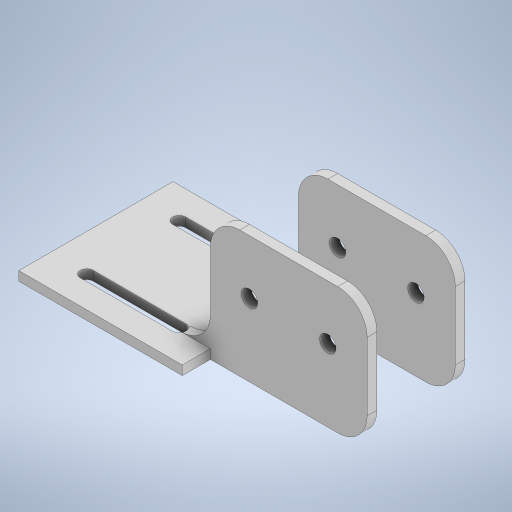
# Autodesk Inventor part: Motor Mount
Saved by Autodesk Inventor 2024 (Build 280153000, 153)
## iProperties
Created: 2024-01-25
Part Number: Motor Mount
Material: Generic
Document SubType Name: Modeling
Designer: aidan
Density: 1 g/cm^3
Appearance: Default
Author: aidan
Autodesk Inventor part; units mm, degrees
ref_plane "YZ Plane" through (0, 0, 0) normal (1, 0, 0) x (0, 1, 0)
ref_plane "XZ Plane" through (0, 0, 0) normal (0, 1, 0) x (-1, 0, 0)
ref_plane "XY Plane" through (0, 0, 0) normal (0, 0, 1) x (1, 0, 0)
sketch "Sketch1" plane through (0, 0, 0) normal (0, 1, 0) x (-1, 0, 0)
  line L0 (0, 0) -> (52.9999, 0)
  line L1 (52.9999, 0) -> (52.9999, 49.9999)
  line L2 (52.9999, 49.9999) -> (0, 49.9999)
  line L3 (0, 49.9999) -> (0, 0)
  dimension "d0" = 52.9999
  dimension "d1" = 49.9999
  constraints: 8 end point, 2 parallel, 1 horizontal, 1 perpendicular
  measures "d0" distance of L1.end L2.end
  measures "d1" distance of L0.end L1.end
extrude "Extrusion1" add sketch "Sketch1" along normal blind 3
sketch "Sketch2" plane through (0, 3, 0) normal (0, 1, 0) x (1, 0, 0)
  line L0 (-52.9999, 0) -> (-52.9999, -49.9999) projected
  line L1 (0, 0) -> (-52.9999, 0) projected
  line L2 (-52.9999, -49.9999) -> (-49.9999, -49.9999)
  line L3 (-49.9999, -49.9999) -> (-49.9999, 0)
  line L4 (-49.9999, 0) -> (-52.9999, 0)
  line L5 (-52.9999, 0) -> (-52.9999, -49.9999)
  dimension "d4" = 3
  constraints: 8 end point, 2 parallel, 1 horizontal, 1 perpendicular, 1 point on line
  measures "d4" distance of L0.end L2.end
extrude "Extrusion2" add sketch "Sketch2" along normal blind 50.9999
sketch "Sketch3" plane through (0, 3, 0) normal (0, 1, 0) x (1, 0, 0)
  line L0 (0, -49.9999) -> (0, 0) projected
  line L1 (0, -10.0051) -> (-11, -10.0051)
  circle A0 centre (-11, -10.0051) radius 2.1
  line L2 (-11, -10.0051) -> (-40.9999, -10.0051)
  circle A1 centre (-40.9999, -10.0051) radius 2.0955
  line L3 (-41.0003, -12.1006) -> (-11.0003, -12.1051)
  line L4 (-11.0003, -7.9051) -> (-41.0003, -7.9096)
  line L5 (0, -40.005) -> (-10.9982, -40.005)
  circle A2 centre (-10.9982, -40.005) radius 2.0955
  circle A3 centre (-41.0003, -40.005) radius 2.0955
  line L6 (-41.0003, -42.1005) -> (-10.9982, -42.1005)
  line L7 (-10.9982, -37.9095) -> (-41.0003, -37.9095)
  line L8 (-49.9999, -49.9999) -> (0, -49.9999) projected
  line L9 (0, 0) -> (-49.9999, 0) projected
  dimension "d7" = 11
  dimension "d8" = 4.2
  dimension "d9" = 29.9999
  dimension "d10" = 4.191
  dimension "d11" = 10.9982
  dimension "d12" = 4.191
  dimension "d13" = 4.191
  dimension "d14" = 29.9999
  dimension "d15" = 9.9949
  dimension "d16" = 10.0051
  constraints: 14 end point, 8 point on circle, 4 centre point, 3 coincident, 3 horizontal, 3 tangent, 2 point on line, 1 perpendicular
  measures "d7" distance of L1.start L1.end
  measures "d8" diameter of A0
  measures "d9" distance of L2.start L2.end
  measures "d10" diameter of A1
  measures "d11" distance of L5.start L5.end
  measures "d12" diameter of A2
  measures "d13" diameter of A3
  measures "d14" distance of L1.end L5.end
  measures "d15" distance between parallel lines of L8 L5
  measures "d16" distance between parallel lines of L9 L1
extrude "Extrusion3" cut sketch "Sketch3" against normal blind 12.5001
sketch "Sketch4" plane through (-49.9999, 3, 49.9999) normal (1, 0, 0) x (0, 0, -1)
  line L0 (0, 0) -> (75.0771, 0)
  line L1 (75.0771, 0) -> (75.0771, 61.4619)
  line L2 (75.0771, 61.4619) -> (0, 61.4619)
  line L3 (0, 61.4619) -> (0, 0)
  point P0 (49.9999, -3)
  constraints: 8 end point, 2 parallel, 1 horizontal, 1 perpendicular
extrude "Extrusion4" cut sketch "Sketch4" against normal blind 22.225
sketch "Sketch5" plane through (0, 3, 0) normal (0, 1, 0) x (1, 0, 0)
  line L0 (0, -49.9999) -> (0, 0) projected
  line L1 (0, -37.6809) -> (-52.8078, -37.6809)
  line L2 (-52.8078, -37.6809) -> (-52.8078, -40.8559)
  line L3 (-52.8078, -40.8559) -> (0, -40.8559)
  line L4 (0, -40.8559) -> (0, -37.6809)
  line L5 (-52.9999, -49.9999) -> (-52.9999, 0) projected
  line L6 (0, -12.2809) -> (-52.9999, -12.2809)
  line L7 (-52.9999, -12.2809) -> (-52.9999, -9.1059)
  line L8 (-52.9999, -9.1059) -> (0, -9.1059)
  line L9 (0, -9.1059) -> (0, -12.2809)
  line L10 (-52.9999, -49.9999) -> (0, -49.9999) projected
  point P0 (0, -9.1059)
  point P1 (0, -40.8559)
  dimension "d21" = 3.175
  dimension "d22" = 3.175
  dimension "d23" = 25.4
  dimension "d24" = 9.144
  constraints: 16 end point, 4 parallel, 3 point on line, 2 horizontal, 2 perpendicular
  measures "d21" distance between parallel lines of L8 L6
  measures "d22" distance between parallel lines of L3 L1
  measures "d23" distance between parallel lines of L6 L1
  measures "d24" distance between parallel lines of L10 L3
extrude "Extrusion5" add sketch "Sketch5" along normal blind 42.3418 contours L3 L2 L1 L0 | L5 L8 L0 L6
sketch "Sketch6" plane through (-42.9152, 3, 40.8559) normal (0, 0, 1) x (1, 0, 0)
  line L0 (-10.0847, 0) -> (0.0225, 0) projected
  line L1 (-10.0847, 0) -> (60.9506, 0)
  line L2 (60.9506, 0) -> (60.9506, 16.9418)
  line L3 (60.9506, 16.9418) -> (-10.0847, 16.9418)
  line L4 (-10.0847, 16.9418) -> (-10.0847, 0)
  point P0 (42.9152, -3)
  dimension "d27" = 16.9418
  constraints: 8 end point, 2 parallel, 1 horizontal, 1 perpendicular
  measures "d27" distance of L1.end L2.end
extrude "Extrusion6" cut sketch "Sketch6" against normal blind 32.2707
sketch "Sketch7" plane through (-52.9999, 0, 49.9999) normal (0, 0, 1) x (1, 0, 0)
  line L0 (0, 3) -> (52.9999, 3) projected
  line L1 (0, 0) -> (0, 3) projected
  line L2 (0, 0) -> (52.9999, 0) projected
  line L3 (52.9999, 0) -> (52.9999, 3) projected
  point P0 (52.9999, 0)
extrude "Extrusion7" add sketch "Sketch7" along normal blind 3.175
sketch "Sketch8" plane through (0, 3, 0) normal (0, 1, 0) x (1, 0, 0)
  line L0 (0, -53.1749) -> (-52.9999, -53.1749) projected
  line L1 (-52.9999, -53.1749) -> (0, -53.1749)
  line L2 (0, -53.1749) -> (0, -49.9999)
  line L3 (0, -49.9999) -> (-52.9999, -49.9999)
  line L4 (-52.9999, -49.9999) -> (-52.9999, -53.1749)
  point P0 (0, 0)
  dimension "d32" = 3.175
  constraints: 8 end point, 2 parallel, 1 horizontal, 1 perpendicular
  measures "d32" distance between parallel lines of L0 L3
extrude "Extrusion8" add sketch "Sketch8" along normal blind 25.4
sketch "Sketch9" plane through (0, 3, 49.9999) normal (0, 0, -1) x (-1, 0, 0)
  line L0 (52.9999, 0) -> (52.9999, 25.4) projected
  line L1 (0, 0) -> (0, 25.4) projected
  line L2 (52.9999, 25.4) -> (0, 25.4)
  line L3 (0, 25.4) -> (0, 16.764)
  line L4 (0, 16.764) -> (52.9999, 16.764)
  line L5 (52.9999, 16.764) -> (52.9999, 25.4)
  point P0 (0, -3)
  point P1 (52.9999, 16.764)
  dimension "d35" = 8.636
  constraints: 8 end point, 2 parallel, 1 horizontal, 1 perpendicular, 1 point on line
  measures "d35" distance between parallel lines of L4 L2
extrude "Extrusion9" add sketch "Sketch9" along normal blind 11.1125
sketch "Sketch10" plane through (-52.9999, 0, 53.1749) normal (0, 0, 1) x (1, 0, 0)
  line L0 (0.1921, 19.9418) -> (0.1921, 45.3418) projected
  line L1 (0.1921, 28.4) -> (52.9999, 28.4) projected
  line L2 (0.1921, 45.3418) -> (52.9999, 45.3418)
  line L3 (52.9999, 45.3418) -> (52.9999, 28.4)
  line L4 (52.9999, 28.4) -> (0.1921, 28.4)
  line L5 (0.1921, 28.4) -> (0.1921, 45.3418)
  point P0 (52.9999, 0)
  constraints: 8 end point, 2 parallel, 1 horizontal, 1 perpendicular
extrude "Extrusion10" cut sketch "Sketch10" against normal blind 74.6125
sketch "Sketch11" plane through (-52.9999, 45.3418, 9.1059) normal (-1, 0, 0) x (0, 0, 1)
  line L0 (0, -25.4) -> (0, 0) projected
  line L1 (0, -25.4) -> (3.175, -25.4) projected
  line L2 (3.175, -25.4) -> (3.175, 0) projected
  line L3 (0, 0) -> (3.175, 0) projected
  line L4 (0, -25.4) -> (0, 0) projected
  line L5 (-9.1059, -42.3418) -> (40.894, -42.3418) projected
  line L6 (-9.1059, -45.3418) -> (-9.1059, -42.3418) projected
  line L7 (-9.1059, -45.3418) -> (44.069, -45.3418) projected
  line L8 (44.069, -45.3418) -> (44.069, -16.9418) projected
  line L9 (44.069, -16.9418) -> (29.7815, -16.9418) projected
  line L10 (29.7815, -25.5778) -> (29.7815, -16.9418) projected
  line L11 (40.894, -25.5778) -> (29.7815, -25.5778) projected
  line L12 (40.894, -42.3418) -> (40.894, -25.5778) projected
  line L13 (46.1792, -25.5778) -> (63.7635, -25.5778)
  line L14 (63.7635, -25.5778) -> (63.7635, -15.0041)
  line L15 (63.7635, -15.0041) -> (46.1792, -15.0041)
  line L16 (46.1792, -15.0041) -> (46.1792, -25.5778)
  line L17 (46.1792, -15.0041) -> (20.9984, -15.0041)
  line L18 (20.9984, -15.0041) -> (20.9984, -26.5395)
  line L19 (20.9984, -26.5395) -> (46.1792, -26.5395)
  line L20 (46.1792, -26.5395) -> (46.1792, -15.0041)
  point P0 (-9.1059, -45.3418)
  constraints: 16 end point, 4 parallel, 2 horizontal, 2 perpendicular
extrude "Extrusion11" cut sketch "Sketch11" against normal blind 84.1375 contours L0 L3 L2 L1 | L19 L18 L17 L16 L20 L8 L9 L10 L11 L12 | L12 L11 L10 L9 L8 L19 | L15 L14 L13 L16
sketch "Sketch12" plane through (0, 0, 0) normal (0, -1, 0) x (1, 0, 0)
  line L0 (-52.9999, 49.9999) -> (0, 49.9999) projected
  line L1 (-52.9999, 49.9999) -> (0, 49.9999)
  line L2 (0, 49.9999) -> (0, 57.3175)
  line L3 (0, 57.3175) -> (-52.9999, 57.3175)
  line L4 (-52.9999, 57.3175) -> (-52.9999, 49.9999)
  point P0 (0, 0)
  constraints: 8 end point, 2 parallel, 1 horizontal, 1 perpendicular
extrude "Extrusion12" cut sketch "Sketch12" against normal blind 52.3875
sketch "Sketch13" plane through (0, 3, 0) normal (0, 1, 0) x (1, 0, 0)
  line L0 (-11.0003, -12.1051) -> (-41.0003, -12.1006) projected
  line L1 (-41.0003, -37.9095) -> (-10.9982, -37.9095) projected
  line L2 (-11.0003, -12.1051) -> (-41.0003, -12.1051)
  line L3 (-41.0003, -12.1051) -> (-41.0003, -37.9095)
  line L4 (-41.0003, -37.9095) -> (-11.0003, -37.9095)
  line L5 (-11.0003, -37.9095) -> (-11.0003, -12.1051)
  line L6 (-41.0003, -37.9095) -> (-41.0003, -12.1051)
  line L7 (-11.0003, -37.9095) -> (0, -37.9095)
  line L8 (0, -37.9095) -> (0, -12.1051)
  line L9 (0, -12.1051) -> (-11.0003, -12.1051)
  line L10 (-11.0003, -12.1051) -> (-11.0003, -37.9095)
  line L11 (-52.9999, 0) -> (-52.9999, -49.9999) projected
  line L12 (-52.9999, -12.1051) -> (-41.0003, -12.1051)
  line L13 (-41.0003, -12.1051) -> (-41.0003, -37.9095)
  line L14 (-41.0003, -37.9095) -> (-52.9999, -37.9095)
  line L15 (-52.9999, -37.9095) -> (-52.9999, -12.1051)
  point P0 (0, 0)
  point P1 (-10.9982, -37.9095)
  constraints: 26 end point, 6 parallel, 3 horizontal, 3 perpendicular, 1 point on line
extrude "Extrusion13" add sketch "Sketch13" along normal blind 10.795
sketch "Sketch14" plane through (-11.0003, 3, 12.1051) normal (0, 0, -1) x (-1, 0, 0)
  line L0 (41.9996, 0) -> (41.9996, 10.795) projected
  line L1 (41.9996, 5.3975) -> (29.2996, 5.3975)
  line L2 (29.2996, 5.3975) -> (3.8996, 5.3975)
  circle A0 centre (29.2996, 5.3975) radius 2.6289
  circle A1 centre (3.8996, 5.3975) radius 2.6289
  point P0 (-11.0003, -3)
  dimension "d46" = 12.7
  dimension "d47" = 25.4
  dimension "d48" = 5.2578
  dimension "d49" = 5.2578
  constraints: 4 end point, 2 centre point, 2 coincident, 2 horizontal, 1 midpoint
  measures "d46" distance of L1.start L1.end
  measures "d47" distance of L1.end L2.end
  measures "d48" diameter of A0
  measures "d49" diameter of A1
extrude "Extrusion14" cut sketch "Sketch14" against normal blind 40.005
sketch "Sketch15" plane through (0, 13.795, 0) normal (0, 1, 0) x (1, 0, 0)
  line L0 (0, -12.1051) -> (-52.9999, -12.1051) projected
  line L1 (-52.9999, -12.1051) -> (-52.9999, -37.9095) projected
  line L2 (-52.9999, -37.9095) -> (0, -37.9095) projected
  line L3 (0, -37.9095) -> (0, -12.1051) projected
  point P0 (0, 0)
extrude "Extrusion15" cut sketch "Sketch15" against normal blind 10.795
sketch "Sketch16" plane through (0, 0, 0) normal (1, 0, 0) x (0, 0, -1)
  line L0 (0, 0) -> (-49.9999, 0) projected
  line L1 (0, 3) -> (-49.9999, 3) projected
  line L2 (-12.3063, 0) -> (-37.7063, 0)
  line L3 (-37.7063, 0) -> (-37.7063, 3)
  line L4 (-37.7063, 3) -> (-12.3063, 3)
  line L5 (-12.3063, 3) -> (-12.3063, 0)
  line L6 (0, 0) -> (0, 3) projected
  line L7 (-49.9999, 3) -> (-49.9999, 0) projected
  line L8 (-12.3063, 3) -> (-9.1313, 3)
  line L9 (-9.1313, 3) -> (-9.1313, 0)
  line L10 (-9.1313, 0) -> (-12.3063, 0)
  line L11 (-12.3063, 0) -> (-12.3063, 3)
  line L12 (-37.7063, 3) -> (-40.8813, 3)
  line L13 (-40.8813, 3) -> (-40.8813, 0)
  line L14 (-40.8813, 0) -> (-37.7063, 0)
  line L15 (-37.7063, 0) -> (-37.7063, 3)
  point P0 (0, 1.5)
  point P1 (-12.3063, 3)
  dimension "d54" = 25.4
  dimension "d55" = 12.3063
  dimension "d56" = 12.2936
  dimension "d57" = 3.175
  dimension "d58" = 3.175
  constraints: 24 end point, 6 parallel, 4 point on line, 3 horizontal, 3 perpendicular, 1 midpoint
  measures "d54" distance between parallel lines of L3 L5
  measures "d55" distance from line of point (0, 1.5) L5
  measures "d56" distance between parallel lines of L3 L7
  measures "d57" distance of L9.end L10.end
  measures "d58" distance of L14.end L13.end
extrude "Extrusion16" add sketch "Sketch16" along normal blind 25.4 contours L0 L5 L1 L9 | L0 L13 L1 L3
sketch "Sketch17" plane through (0, 3, 0) normal (0, 1, 0) x (1, 0, 0)
  line L0 (0, 0) -> (0, -9.1313) projected
  line L1 (0, -12.3063) -> (25.4, -12.3063) projected
  line L2 (0, -9.1313) -> (25.4, -9.1313)
  line L3 (25.4, -9.1313) -> (25.4, -12.3063)
  line L4 (25.4, -12.3063) -> (0, -12.3063)
  line L5 (0, -12.3063) -> (0, -9.1313)
  line L6 (0, -37.7063) -> (25.4, -37.7063) projected
  line L7 (0, -40.8813) -> (25.4, -40.8813) projected
  line L8 (25.4, -37.7063) -> (0, -37.7063)
  line L9 (0, -37.7063) -> (0, -40.8813)
  line L10 (0, -40.8813) -> (25.4, -40.8813)
  line L11 (25.4, -40.8813) -> (25.4, -37.7063)
  constraints: 16 end point, 4 parallel, 2 horizontal, 2 perpendicular
extrude "Extrusion17" add sketch "Sketch17" along normal blind 38.1
fillet "Fillet1" radius 9.525 2 edges at (0, 3, 10.7188) (0, 3, 39.2938)
sketch "Sketch18" plane through (0, 0, 0) normal (0, -1, 0) x (1, 0, 0)
  point P0 (25.4, 9.1313)
  point P1 (25.4, 37.7063)
sketch "Sketch19" plane through (0, 0, 9.1313) normal (0, 0, -1) x (-1, 0, 0)
  line L0 (0, 41.1) -> (-25.4, 41.1) projected
  line L1 (-12.7, 41.1) -> (-12.7, 28.4)
  line L2 (-12.7, 28.4) -> (-12.7, 3)
  circle A0 centre (-12.7, 28.4) radius 2.6289
  circle A1 centre (-12.7, 8.7553) radius 2.6289
  point P0 (0, 0)
  dimension "d64" = 12.7
  dimension "d65" = 25.4
  dimension "d66" = 5.2578
  dimension "d67" = 5.2578
  constraints: 4 end point, 2 centre point, 2 point on line, 1 coincident, 1 midpoint, 1 vertical
  measures "d64" distance of L1.start L1.end
  measures "d65" distance of L1.end L2.end
  measures "d66" diameter of A0
  measures "d67" diameter of A1
extrude "Extrusion18" cut sketch "Sketch19" against normal blind 198.4375
sketch "Sketch20" plane through (0, 0, 40.8813) normal (0, 0, 1) x (1, 0, 0)
  line L0 (0, 0) -> (25.4, 0) projected
  line L1 (12.7, 0) -> (12.7, 10.795)
  line L2 (12.7, 10.795) -> (12.7, 23.495)
  circle A0 centre (12.7, 23.495) radius 2.6289
  dimension "d70" = 10.795
  dimension "d71" = 12.7
  dimension "d72" = 5.2578
  constraints: 4 end point, 2 vertical, 1 centre point, 1 coincident, 1 midpoint
  measures "d70" distance of L1.start L1.end
  measures "d71" distance of L1.end L2.end
  measures "d72" diameter of A0
sketch "Sketch21" plane through (0, 0, 40.8813) normal (0, 0, 1) x (1, 0, 0)
  circle A0 centre (12.7, 8.7553) radius 2.6289 projected
  circle A1 centre (12.7, 28.4) radius 2.6289 projected
  circle A2 centre (12.7, 28.4) radius 2.6289 projected
  circle A3 centre (12.7, 8.7553) radius 2.6289 projected
  circle A4 centre (12.7, 28.4) radius 2.6289 projected
  point P0 (0, 0)
extrude "Extrusion19" add sketch "Sketch21" against normal blind 3.175
sketch "Sketch22" plane through (0, 0, 9.1313) normal (0, 0, -1) x (-1, 0, 0)
  circle A0 centre (-12.7, 28.4) radius 2.6289 projected
  circle A1 centre (-12.7, 8.7553) radius 2.6289 projected
  point P0 (0, 0)
extrude "Extrusion20" add sketch "Sketch22" against normal blind 3.175
extrude "Extrusion21" cut sketch "Sketch20" against normal blind 47.625
fillet "Fillet2" radius 9.525 2 edges at (0, 41.1, 10.7188) (0, 41.1, 39.2938)
sketch "Sketch23" plane through (0, 0, 40.8813) normal (0, 0, 1) x (1, 0, 0)
  circle A0 centre (12.7, 23.495) radius 2.6289 projected
  line L0 (12.7, 23.495) -> (38.1, 23.495)
  circle A1 centre (38.1, 23.495) radius 2.6289
  point P0 (0, 0)
  dimension "d80" = 25.4
  dimension "d81" = 5.2578
  constraints: 2 end point, 1 centre point, 1 coincident, 1 horizontal
  measures "d80" distance of L0.start L0.end
  measures "d81" diameter of A1
sketch "Sketch24" plane through (25.4, 0, 0) normal (1, 0, 0) x (0, 0, -1)
  line L0 (-40.8813, 0) -> (-37.7063, 0) projected
  line L1 (-37.7063, 0) -> (-37.7063, 41.1) projected
  line L2 (-40.8813, 41.1) -> (-37.7063, 41.1) projected
  line L3 (-40.8813, 0) -> (-40.8813, 41.1) projected
  line L4 (-12.3063, 0) -> (-12.3063, 41.1) projected
  line L5 (-12.3063, 0) -> (-9.1313, 0) projected
  line L6 (-9.1313, 0) -> (-9.1313, 41.1) projected
  line L7 (-12.3063, 41.1) -> (-9.1313, 41.1) projected
  point P0 (0, 0)
extrude "Extrusion22" add sketch "Sketch24" along normal blind 25.4
extrude "Extrusion23" cut sketch "Sketch23" against normal blind 36.5125 contours A1
fillet "Fillet3" radius 9.525 4 edges at (50.8, 41.1, 39.2938) (50.8, 41.1, 10.7188) (50.8, 0, 10.7188) (50.8, 0, 39.2938)
body "Solid1"
